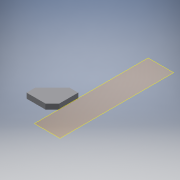
# Autodesk Inventor part: Gusset
Saved by Autodesk Inventor 2018 (Build 220112000, 112)
## iProperties
Created: 2018-05-29
Part Number: Gusset
Material: Steel, Alloy
Document SubType Name: Modeling
Designer: P136265
Mass: 82.5564 g
Surface Area: 35.3635 cm^2
Volume: 10.68 cm^3
Density: 7.73 g/cm^3
Appearance: Semi-Polished
Author: P136265
Autodesk Inventor part; units mm, degrees
ref_plane "YZ Plane" through (0, 0, 0) normal (1, 0, 0) x (0, 1, 0)
ref_plane "XZ Plane" through (0, 0, 0) normal (0, 1, 0) x (-1, 0, 0)
ref_plane "XY Plane" through (0, 0, 0) normal (0, 0, 1) x (1, 0, 0)
ref_plane "Work Plane1" through (0, 0, -17.5) normal (0, 0, 1) x (1, 0, 0)
sketch "Sketch1" plane through (0, 0, -17.5) normal (0, 0, 1) x (1, 0, 0)
  line L0 (-31, 0) -> (-31, 120) construction
  line L1 (3, 17.5) -> (-715, 17.5) construction
  line L2 (-39, 17.5) -> (-81, 17.5)
  line L3 (-81, 17.5) -> (-81, 27.5)
  line L4 (-41, 47.5) -> (-31, 47.5)
  line L5 (-31, 47.5) -> (-31, 25.5)
  line L6 (-31, 25.5) -> (-39, 17.5)
  line L7 (-81, 27.5) -> (-41, 47.5)
  point P0 (0, 0)
  point P1 (-31, 17.5)
  point P2 (-81, 47.5)
  dimension "d0" = 50
  dimension "d1" = 30
  dimension "d2" = 8
  dimension "d3" = 8
  dimension "d4" = 20
  dimension "d5" = 40
  constraints: 12 end point, 6 point on line, 2 parallel, 1 horizontal, 1 perpendicular
  measures "d0" distance of point (-81, 47.5) L4.end
  measures "d1" distance of L2.end point (-81, 47.5)
  measures "d2" distance of L5.end point (-31, 17.5)
  measures "d3" distance of L2.start point (-31, 17.5)
  measures "d4" distance of L3.end point (-81, 47.5)
  measures "d5" distance of L4.start point (-81, 47.5)
extrude "Extrusion1" add sketch "Sketch1" along normal mid plane 10
equation "\"d3\" = d2"
body "Solid1"
